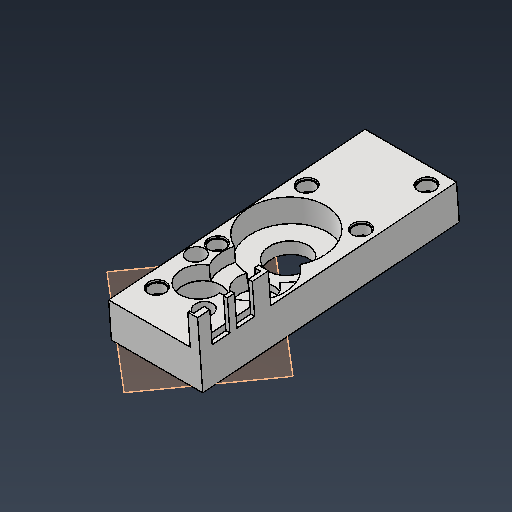
# Autodesk Inventor part: Right_gearbox
Saved by Autodesk Inventor 2026.2 (Build 302298010, 298A)
## iProperties
Created: 2026-04-04
Part Number: Right_gearbox
Material: Generic
Document SubType Name: Modeling
Designer: szymo
Density: 1 g/cm^3
Appearance: Default
Author: szymo
Autodesk Inventor part; units mm, degrees
(part 1 of 2)
ref_plane "YZ Plane" through (0, 0, 0) normal (1, 0, 0) x (0, 1, 0)
ref_plane "XZ Plane" through (0, 0, 0) normal (0, 1, 0) x (-1, 0, 0)
ref_plane "XY Plane" through (0, 0, 0) normal (0, 0, 1) x (1, 0, 0)
ref_plane "Work Plane1" through (-23.709139, -17.243721, 13.989977) normal (0, 0.9970894, 0.0762418) x (-1, 0, 0)
sketch "Sketch1" plane through (-23.709139, -17.243721, 13.989977) normal (0, 0.9970894, 0.0762418) x (-1, 0, 0)
  line L0 (0, -0.624975) -> (23.2, -0.624975)
  line L1 (23.2, -0.624975) -> (23.2, -65.920816)
  line L2 (23.2, -65.920816) -> (0, -65.920816)
  line L3 (0, -65.920816) -> (0, -0.624975)
  circle A0 centre (9.208398, -23.610194) radius 8 construction
  circle A1 centre (13, -35.626174) radius 9.6 construction
  circle A2 centre (9.208398, -23.610194) radius 8.4
  circle A3 centre (13, -35.626174) radius 10
  circle A4 centre (9.208398, -23.610194) radius 4.2 construction
  circle A5 centre (9.208398, -23.610194) radius 4.6
  circle A6 centre (14.459131, -15.124975) radius 1.15
  circle A7 centre (14.459131, -15.124975) radius 5
  circle A8 centre (14.5, -15.124975) radius 13.85 construction
  circle A9 centre (14.5, -55.920816) radius 14.5 construction
  circle A10 centre (14.5, -15.124975) radius 14.5 construction
  line L4 (19.165073, -50.048244) -> (22.270069, -47.442843)
  arc A11 (24.198432, -49.740976) -> (22.270069, -47.442843) centre (14.5, -55.920816) ccw
  line L5 (24.198432, -49.740976) -> (21.093435, -52.346377)
  arc A12 (21.093435, -52.346377) -> (19.165073, -50.048244) centre (14.5, -55.920816) ccw
  arc A13 (4.801568, -62.100655) -> (6.729931, -64.398789) centre (14.5, -55.920816) ccw
  line L6 (4.801568, -62.100655) -> (7.906565, -59.495254)
  arc A14 (7.906565, -59.495254) -> (9.834927, -61.793387) centre (14.5, -55.920816) ccw
  line L7 (9.834927, -61.793387) -> (6.729931, -64.398789)
  circle A15 centre (14.5, -55.920816) radius 5
  circle A16 centre (14.5, -55.920816) radius 13.85
  line L8 (20.703236, -53.979201) -> (25.489059, -49.963418)
  arc A17 (25.489059, -49.963418) -> (22.275121, -46.133196) centre (14.5, -55.920816) ccw
  line L9 (22.275121, -46.133196) -> (17.489298, -50.148979)
  arc A18 (20.703236, -53.979201) -> (17.489298, -50.148979) centre (14.5, -55.920816) ccw
  arc A19 (3.510941, -61.878213) -> (6.724879, -65.708435) centre (14.5, -55.920816) ccw
  line L10 (3.510941, -61.878213) -> (8.296764, -57.86243)
  arc A20 (8.296764, -57.86243) -> (11.510702, -61.692652) centre (14.5, -55.920816) ccw
  line L11 (11.510702, -61.692652) -> (6.724879, -65.708435)
  line L12 (6.724879, -65.708435) -> (6.724879, -65.920816)
  line L13 (11.510702, -61.692652) -> (23.2, -61.692652)
  arc A21 (20.63224, -38.75849) -> (22.059739, -38.801252) centre (21.52446, -32.822118) ccw
  arc A22 (22.059739, -38.801252) -> (22.213494, -38.322751) centre (13, -35.626174) ccw
  arc A23 (22.213494, -38.322751) -> (21.028277, -37.525981) centre (18.295517, -42.87094) ccw
  arc A24 (21.028277, -37.525981) -> (21.116703, -37.10321) centre (13, -35.626174) ccw
  arc A25 (21.116703, -37.10321) -> (22.521898, -36.848243) centre (20.755184, -31.111058) ccw
  arc A26 (22.521898, -36.848243) -> (22.572807, -36.348231) centre (13, -35.626174) ccw
  arc A27 (22.572807, -36.348231) -> (21.247832, -35.815293) centre (19.686069, -41.611625) ccw
  arc A28 (21.247832, -35.815293) -> (21.246426, -35.383375) centre (13, -35.626174) ccw
  arc A29 (21.246426, -35.383375) -> (22.567904, -34.841824) centre (19.64697, -29.597331) ccw
  arc A30 (22.567904, -34.841824) -> (22.513742, -34.342154) centre (13, -35.626174) ccw
  arc A31 (22.513742, -34.342154) -> (21.106917, -34.096339) centre (20.784408, -40.090717) ccw
  arc A32 (21.106917, -34.096339) -> (21.015742, -33.674153) centre (13, -35.626174) ccw
  arc A33 (21.015742, -33.674153) -> (22.195747, -32.869685) centre (18.248251, -28.347093) ccw
  arc A34 (22.195747, -32.869685) -> (22.038882, -32.392195) centre (13, -35.626174) ccw
  arc A35 (22.038882, -32.392195) -> (20.611691, -32.444247) centre (21.54253, -38.374686) ccw
  arc A36 (20.611691, -32.444247) -> (20.434731, -32.050243) centre (13, -35.626174) ccw
  arc A37 (20.434731, -32.050243) -> (21.421692, -31.018018) centre (16.620158, -27.414986) ccw
  arc A38 (21.421692, -31.018018) -> (21.168978, -30.583576) centre (13, -35.626174) ccw
  arc A39 (21.168978, -30.583576) -> (19.783798, -30.93122) centre (21.927304, -36.538533) ccw
  arc A40 (19.783798, -30.93122) -> (19.528786, -30.582618) centre (13, -35.626174) ccw
  arc A41 (19.528786, -30.582618) -> (20.279568, -29.367749) centre (14.833847, -26.841747) ccw
  arc A42 (20.279568, -29.367749) -> (19.942051, -28.995342) centre (13, -35.626174) ccw
  arc A43 (19.942051, -28.995342) -> (18.65942, -29.623385) centre (21.921911, -34.662505) ccw
  arc A44 (18.65942, -29.623385) -> (18.337502, -29.335421) centre (13, -35.626174) ccw
  arc A45 (18.337502, -29.335421) -> (18.819293, -27.991003) centre (12.967388, -26.652429) ccw
  arc A46 (18.819293, -27.991003) -> (18.411724, -27.696908) centre (13, -35.626174) ccw
  arc A47 (18.411724, -27.696908) -> (17.287698, -28.577901) centre (21.526587, -32.828594) ccw
  arc A48 (17.287698, -28.577901) -> (16.912944, -28.36316) centre (13, -35.626174) ccw
  arc A49 (16.912944, -28.36316) -> (17.104686, -26.947951) centre (11.102354, -26.855308) ccw
  arc A50 (17.104686, -26.947951) -> (16.644878, -26.745021) centre (13, -35.626174) ccw
  arc A51 (16.644878, -26.745021) -> (15.728583, -27.84046) centre (20.758611, -31.11695) ccw
  arc A52 (15.728583, -27.84046) -> (15.317371, -27.708327) centre (13, -35.626174) ccw
  arc A53 (15.317371, -27.708327) -> (15.210685, -26.284178) centre (9.320257, -27.441515) ccw
  arc A54 (15.210685, -26.284178) -> (14.718733, -26.181283) centre (13, -35.626174) ccw
  arc A55 (14.718733, -26.181283) -> (14.050216, -27.443292) centre (19.651547, -29.602382) ccw
  arc A56 (14.050216, -27.443292) -> (13.620518, -27.399543) centre (13, -35.626174) ccw
  arc A57 (13.620518, -27.399543) -> (13.220066, -26.028696) centre (7.698982, -28.385431) ccw
  arc A58 (13.220066, -26.028696) -> (12.717471, -26.030332) centre (13, -35.626174) ccw
  arc A59 (12.717471, -26.030332) -> (12.32595, -27.403756) centre (18.253778, -28.351081) ccw
  arc A60 (12.32595, -27.403756) -> (11.896546, -27.450301) centre (13, -35.626174) ccw
  arc A61 (11.896546, -27.450301) -> (11.219829, -26.19267) centre (6.309387, -29.645802) ccw
  arc A62 (11.219829, -26.19267) -> (10.728557, -26.298765) centre (13, -35.626174) ccw
  arc A63 (10.728557, -26.298765) -> (10.631143, -27.723578) centre (16.626394, -27.417738) ccw
  arc A64 (10.631143, -27.723578) -> (10.220799, -27.858385) centre (13, -35.626174) ccw
  arc A65 (10.220799, -27.858385) -> (9.297395, -26.768933) centre (5.212203, -31.167544) ccw
  arc A66 (9.297395, -26.768933) -> (8.838917, -26.974851) centre (13, -35.626174) ccw
  arc A67 (8.838917, -26.974851) -> (9.039866, -28.388782) centre (14.840518, -26.843142) ccw
  arc A68 (9.039866, -28.388782) -> (8.666517, -28.605958) centre (13, -35.626174) ccw
  arc A69 (8.666517, -28.605958) -> (7.536781, -27.7323) centre (4.455384, -32.88415) ccw
  arc A70 (7.536781, -27.7323) -> (7.131135, -28.029041) centre (13, -35.626174) ccw
  arc A71 (7.131135, -28.029041) -> (7.621666, -29.370294) centre (12.974204, -26.652407) ccw
  arc A72 (7.621666, -29.370294) -> (7.301629, -29.660348) centre (13, -35.626174) ccw
  arc A73 (7.301629, -29.660348) -> (6.014937, -29.040667) centre (4.072006, -34.720595) ccw
  arc A74 (6.014937, -29.040667) -> (5.679851, -29.415262) centre (13, -35.626174) ccw
  arc A75 (5.679851, -29.415262) -> (6.438525, -30.625219) centre (11.109017, -26.853869) ccw
  arc A76 (6.438525, -30.625219) -> (6.185788, -30.975474) centre (13, -35.626174) ccw
  arc A77 (6.185788, -30.975474) -> (4.798374, -30.636852) centre (4.078824, -36.596619) ccw
  arc A78 (4.798374, -30.636852) -> (4.548493, -31.07293) centre (13, -35.626174) ccw
  arc A79 (4.548493, -31.07293) -> (5.542152, -32.098709) centre (9.326474, -27.438722) ccw
  arc A80 (5.542152, -32.098709) -> (5.36776, -32.493857) centre (13, -35.626174) ccw
  arc A81 (5.36776, -32.493857) -> (3.940261, -32.451095) centre (4.47554, -38.430229) ccw
  arc A82 (3.940261, -32.451095) -> (3.786506, -32.929596) centre (13, -35.626174) ccw
  arc A83 (3.786506, -32.929596) -> (4.971723, -33.726366) centre (7.704483, -28.381407) ccw
  arc A84 (4.971723, -33.726366) -> (4.883297, -34.149138) centre (13, -35.626174) ccw
  arc A85 (4.883297, -34.149138) -> (3.478102, -34.404104) centre (5.244816, -40.141289) ccw
  arc A86 (3.478102, -34.404104) -> (3.427193, -34.904116) centre (13, -35.626174) ccw
  arc A87 (3.427193, -34.904116) -> (4.752168, -35.437054) centre (6.313931, -29.640722) ccw
  arc A88 (4.752168, -35.437054) -> (4.753574, -35.868972) centre (13, -35.626174) ccw
  arc A89 (4.753574, -35.868972) -> (3.432096, -36.410523) centre (6.35303, -41.655016) ccw
  arc A90 (3.432096, -36.410523) -> (3.486258, -36.910193) centre (13, -35.626174) ccw
  arc A91 (3.486258, -36.910193) -> (4.893083, -37.156008) centre (5.215592, -31.161631) ccw
  arc A92 (4.893083, -37.156008) -> (4.984258, -37.578194) centre (13, -35.626174) ccw
  arc A93 (4.984258, -37.578194) -> (3.804253, -38.382662) centre (7.751749, -42.905254) ccw
  arc A94 (3.804253, -38.382662) -> (3.961118, -38.860153) centre (13, -35.626174) ccw
  arc A95 (3.961118, -38.860153) -> (5.388309, -38.8081) centre (4.45747, -32.877661) ccw
  arc A96 (5.388309, -38.8081) -> (5.565269, -39.202104) centre (13, -35.626174) ccw
  arc A97 (5.565269, -39.202104) -> (4.578308, -40.234329) centre (9.379842, -43.837361) ccw
  arc A98 (4.578308, -40.234329) -> (4.831022, -40.668771) centre (13, -35.626174) ccw
  arc A99 (4.831022, -40.668771) -> (6.216202, -40.321127) centre (4.072696, -34.713814) ccw
  arc A100 (6.216202, -40.321127) -> (6.471214, -40.669729) centre (13, -35.626174) ccw
  arc A101 (6.471214, -40.669729) -> (5.720432, -41.884598) centre (11.166153, -44.4106) ccw
  arc A102 (5.720432, -41.884598) -> (6.057949, -42.257005) centre (13, -35.626174) ccw
  arc A103 (6.057949, -42.257005) -> (7.34058, -41.628962) centre (4.078089, -36.589842) ccw
  arc A104 (7.34058, -41.628962) -> (7.662498, -41.916926) centre (13, -35.626174) ccw
  arc A105 (7.662498, -41.916926) -> (7.180707, -43.261344) centre (13.032612, -44.599918) ccw
  arc A106 (7.180707, -43.261344) -> (7.588276, -43.555439) centre (13, -35.626174) ccw
  arc A107 (7.588276, -43.555439) -> (8.712302, -42.674446) centre (4.473413, -38.423753) ccw
  arc A108 (8.712302, -42.674446) -> (9.087056, -42.889187) centre (13, -35.626174) ccw
  arc A109 (9.087056, -42.889187) -> (8.895314, -44.304396) centre (14.897646, -44.397039) ccw
  arc A110 (8.895314, -44.304396) -> (9.355122, -44.507326) centre (13, -35.626174) ccw
  arc A111 (9.355122, -44.507326) -> (10.271417, -43.411887) centre (5.241389, -40.135397) ccw
  arc A112 (10.271417, -43.411887) -> (10.682629, -43.54402) centre (13, -35.626174) ccw
  arc A113 (10.682629, -43.54402) -> (10.789315, -44.968169) centre (16.679743, -43.810832) ccw
  arc A114 (10.789315, -44.968169) -> (11.281267, -45.071064) centre (13, -35.626174) ccw
  arc A115 (11.281267, -45.071064) -> (11.949784, -43.809055) centre (6.348453, -41.649966) ccw
  arc A116 (11.949784, -43.809055) -> (12.379482, -43.852804) centre (13, -35.626174) ccw
  arc A117 (12.379482, -43.852804) -> (12.779934, -45.223651) centre (18.301018, -42.866916) ccw
  arc A118 (12.779934, -45.223651) -> (13.282529, -45.222015) centre (13, -35.626174) ccw
  arc A119 (13.282529, -45.222015) -> (13.67405, -43.848591) centre (7.746222, -42.901266) ccw
  arc A120 (13.67405, -43.848591) -> (14.103454, -43.802046) centre (13, -35.626174) ccw
  arc A121 (14.103454, -43.802046) -> (14.780171, -45.059677) centre (19.690613, -41.606545) ccw
  arc A122 (14.780171, -45.059677) -> (15.271443, -44.953582) centre (13, -35.626174) ccw
  arc A123 (15.271443, -44.953582) -> (15.368857, -43.528769) centre (9.373606, -43.834609) ccw
  arc A124 (15.368857, -43.528769) -> (15.779201, -43.393962) centre (13, -35.626174) ccw
  arc A125 (15.779201, -43.393962) -> (16.702605, -44.483414) centre (20.787797, -40.084803) ccw
  arc A126 (16.702605, -44.483414) -> (17.161083, -44.277496) centre (13, -35.626174) ccw
  arc A127 (17.161083, -44.277496) -> (16.960134, -42.863565) centre (11.159482, -44.409205) ccw
  arc A128 (16.960134, -42.863565) -> (17.333483, -42.646389) centre (13, -35.626174) ccw
  arc A129 (17.333483, -42.646389) -> (18.463219, -43.520047) centre (21.544616, -38.368197) ccw
  arc A130 (18.463219, -43.520047) -> (18.868865, -43.223306) centre (13, -35.626174) ccw
  arc A131 (18.868865, -43.223306) -> (18.378334, -41.882053) centre (13.025796, -44.59994) ccw
  arc A132 (18.378334, -41.882053) -> (18.698371, -41.591999) centre (13, -35.626174) ccw
  arc A133 (18.698371, -41.591999) -> (19.985063, -42.21168) centre (21.927994, -36.531752) ccw
  arc A134 (19.985063, -42.21168) -> (20.320149, -41.837085) centre (13, -35.626174) ccw
  arc A135 (20.320149, -41.837085) -> (19.561475, -40.627128) centre (14.890983, -44.398478) ccw construction
  arc A136 (19.561475, -40.627128) -> (19.814212, -40.276874) centre (13, -35.626174) ccw
  arc A137 (19.814212, -40.276874) -> (21.201626, -40.615495) centre (21.921176, -34.655728) ccw
  arc A138 (21.201626, -40.615495) -> (21.451507, -40.179417) centre (13, -35.626174) ccw
  arc A139 (21.451507, -40.179417) -> (20.457848, -39.153638) centre (16.673526, -43.813625) ccw
  arc A140 (20.457848, -39.153638) -> (20.63224, -38.75849) centre (13, -35.626174) ccw
  circle A141 centre (13, -35.626174) radius 5
  circle A142 centre (9.208398, -23.610194) radius 1.25
  arc A143 (5.40627, -25.394522) -> (6.808495, -25.147389) centre (5.476375, -21.690633) ccw
  arc A144 (6.808495, -25.147389) -> (7.029671, -25.447488) centre (9.208398, -23.610194) ccw
  arc A145 (7.029671, -25.447488) -> (6.378522, -26.713709) centre (9.937158, -27.743186) ccw
  arc A146 (6.378522, -26.713709) -> (6.807822, -27.056531) centre (9.208398, -23.610194) ccw
  arc A147 (6.807822, -27.056531) -> (7.898619, -26.141395) centre (5.01659, -23.813817) ccw
  arc A148 (7.898619, -26.141395) -> (8.240212, -26.290701) centre (9.208398, -23.610194) ccw
  arc A149 (8.240212, -26.290701) -> (8.309411, -27.712855) centre (11.906019, -26.82509) ccw
  arc A150 (8.309411, -27.712855) -> (8.852607, -27.795097) centre (9.208398, -23.610194) ccw
  arc A151 (8.852607, -27.795097) -> (9.339696, -26.457168) centre (5.679997, -25.88244) ccw
  arc A152 (9.339696, -26.457168) -> (9.710178, -26.415674) centre (9.208398, -23.610194) ccw
  arc A153 (9.710178, -26.415674) -> (10.481183, -27.612696) centre (13.152054, -25.045566) ccw
  arc A154 (10.481183, -27.612696) -> (10.992725, -27.412322) centre (9.208398, -23.610194) ccw
  arc A155 (10.992725, -27.412322) -> (10.745593, -26.010097) centre (7.288836, -27.342217) ccw
  arc A156 (10.745593, -26.010097) -> (11.045692, -25.788921) centre (9.208398, -23.610194) ccw
  arc A157 (11.045692, -25.788921) -> (12.311913, -26.44007) centre (13.34139, -22.881434) ccw
  arc A158 (12.311913, -26.44007) -> (12.654735, -26.01077) centre (9.208398, -23.610194) ccw
  arc A159 (12.654735, -26.01077) -> (11.739599, -24.919974) centre (9.41202, -27.802002) ccw
  arc A160 (11.739599, -24.919974) -> (11.888905, -24.57838) centre (9.208398, -23.610194) ccw
  arc A161 (11.888905, -24.57838) -> (13.311058, -24.509181) centre (12.423294, -20.912574) ccw
  arc A162 (13.311058, -24.509181) -> (13.393301, -23.965986) centre (9.208398, -23.610194) ccw
  arc A163 (13.393301, -23.965986) -> (12.055372, -23.478896) centre (11.480644, -27.138595) ccw
  arc A164 (12.055372, -23.478896) -> (12.013878, -23.108415) centre (9.208398, -23.610194) ccw
  arc A165 (12.013878, -23.108415) -> (13.210899, -22.337409) centre (10.643769, -19.666538) ccw
  arc A166 (13.210899, -22.337409) -> (13.010526, -21.825867) centre (9.208398, -23.610194) ccw
  arc A167 (13.010526, -21.825867) -> (11.608301, -22.073) centre (12.940421, -25.529756) ccw
  arc A168 (11.608301, -22.073) -> (11.387125, -21.772901) centre (9.208398, -23.610194) ccw
  arc A169 (11.387125, -21.772901) -> (12.038273, -20.50668) centre (8.479638, -19.477202) ccw
  arc A170 (12.038273, -20.50668) -> (11.608973, -20.163858) centre (9.208398, -23.610194) ccw
  arc A171 (11.608973, -20.163858) -> (10.518177, -21.078994) centre (13.400206, -23.406572) ccw
  arc A172 (10.518177, -21.078994) -> (10.176584, -20.929688) centre (9.208398, -23.610194) ccw
  arc A173 (10.176584, -20.929688) -> (10.107385, -19.507534) centre (6.510777, -20.395298) ccw
  arc A174 (10.107385, -19.507534) -> (9.564189, -19.425291) centre (9.208398, -23.610194) ccw
  arc A175 (9.564189, -19.425291) -> (9.0771, -20.76322) centre (12.736799, -21.337949) ccw
  arc A176 (9.0771, -20.76322) -> (8.706618, -20.804715) centre (9.208398, -23.610194) ccw
  arc A177 (8.706618, -20.804715) -> (7.935613, -19.607693) centre (5.264742, -22.174823) ccw
  arc A178 (7.935613, -19.607693) -> (7.42407, -19.808067) centre (9.208398, -23.610194) ccw
  arc A179 (7.42407, -19.808067) -> (7.671203, -21.210292) centre (11.12796, -19.878171) ccw
  arc A180 (7.671203, -21.210292) -> (7.371104, -21.431467) centre (9.208398, -23.610194) ccw
  arc A181 (7.371104, -21.431467) -> (6.104883, -20.780319) centre (5.075406, -24.338955) ccw
  arc A182 (6.104883, -20.780319) -> (5.762061, -21.209619) centre (9.208398, -23.610194) ccw
  arc A183 (5.762061, -21.209619) -> (6.677197, -22.300415) centre (9.004776, -19.418387) ccw
  arc A184 (6.677197, -22.300415) -> (6.527891, -22.642008) centre (9.208398, -23.610194) ccw
  arc A185 (6.527891, -22.642008) -> (5.105737, -22.711208) centre (5.993502, -26.307815) ccw
  arc A186 (5.105737, -22.711208) -> (5.023495, -23.254403) centre (9.208398, -23.610194) ccw
  arc A187 (5.023495, -23.254403) -> (6.361424, -23.741493) centre (6.936152, -20.081794) ccw
  arc A188 (6.361424, -23.741493) -> (6.402918, -24.111974) centre (9.208398, -23.610194) ccw
  arc A189 (6.402918, -24.111974) -> (5.205896, -24.882979) centre (7.773027, -27.553851) ccw
  arc A190 (5.205896, -24.882979) -> (5.40627, -25.394522) centre (9.208398, -23.610194) ccw
  circle A191 centre (9.208398, -23.610194) radius 1.25
  arc A192 (17.179273, -22.928177) -> (16.018307, -22.666389) centre (15.506202, -27.642647) ccw
  arc A193 (16.018307, -22.666389) -> (15.959579, -22.311279) centre (9.208398, -23.610194) ccw
  arc A194 (15.959579, -22.311279) -> (16.974447, -21.689654) centre (13.872622, -17.764852) ccw
  arc A195 (16.974447, -21.689654) -> (16.863291, -21.285842) centre (9.208398, -23.610194) ccw
  arc A196 (16.863291, -21.285842) -> (15.673266, -21.271154) centre (16.206974, -26.245141) ccw
  arc A197 (15.673266, -21.271154) -> (15.54199, -20.936014) centre (9.208398, -23.610194) ccw
  arc A198 (15.54199, -20.936014) -> (16.405438, -20.11697) centre (12.555382, -16.92284) ccw
  arc A199 (16.405438, -20.11697) -> (16.212753, -19.745093) centre (9.208398, -23.610194) ccw
  arc A200 (16.212753, -19.745093) -> (15.045679, -19.978146) centre (16.601875, -24.732476) ccw
  arc A201 (15.045679, -19.978146) -> (14.847592, -19.677624) centre (9.208398, -23.610194) ccw
  arc A202 (14.847592, -19.677624) -> (15.521883, -18.696957) centre (11.091863, -16.373097) ccw
  arc A203 (15.521883, -18.696957) -> (15.256092, -18.373268) centre (9.208398, -23.610194) ccw
  arc A204 (15.256092, -18.373268) -> (14.162975, -18.843876) centre (16.673645, -23.170761) ccw
  arc A205 (14.162975, -18.843876) -> (13.906735, -18.591106) centre (9.208398, -23.610194) ccw
  arc A206 (13.906735, -18.591106) -> (14.362399, -17.491675) centre (9.546028, -16.139651) ccw
  arc A207 (14.362399, -17.491675) -> (14.035117, -17.230321) centre (9.208398, -23.610194) ccw
  arc A208 (14.035117, -17.230321) -> (13.063732, -17.917917) centre (16.419148, -21.628251) ccw
  arc A209 (13.063732, -17.917917) -> (12.760538, -17.723945) centre (9.208398, -23.610194) ccw
  arc A210 (12.760538, -17.723945) -> (12.97766, -16.553803) centre (7.985437, -16.232703) ccw
  arc A211 (12.97766, -16.553803) -> (12.603191, -16.366205) centre (9.208398, -23.610194) ccw
  arc A212 (12.603191, -16.366205) -> (11.795993, -17.240738) centre (15.849507, -20.172362) ccw
  arc A213 (11.795993, -17.240738) -> (11.459095, -17.114043) centre (9.208398, -23.610194) ccw
  arc A214 (11.459095, -17.114043) -> (11.428186, -15.924328) centre (6.478294, -16.648187) ccw
  arc A215 (11.428186, -15.924328) -> (11.022897, -15.818687) centre (9.208398, -23.610194) ccw
  arc A216 (11.022897, -15.818687) -> (10.415163, -16.841935) centre (14.989617, -18.866723) ccw
  arc A217 (10.415163, -16.841935) -> (10.059286, -16.788053) centre (9.208398, -23.610194) ccw
  arc A218 (10.059286, -16.788053) -> (9.781697, -15.630763) centre (5.090471, -17.367944) ccw
  arc A219 (9.781697, -15.630763) -> (9.3633, -15.611694) centre (9.208398, -23.610194) ccw
  arc A220 (9.3633, -15.611694) -> (8.981592, -16.738937) centre (13.87706, -17.768396) ccw
  arc A221 (8.981592, -16.738937) -> (8.622289, -16.760224) centre (9.208398, -23.610194) ccw
  arc A222 (8.622289, -16.760224) -> (8.110152, -15.685937) centre (3.882621, -18.360517) ccw
  arc A223 (8.110152, -15.685937) -> (7.696933, -15.754275) centre (9.208398, -23.610194) ccw
  arc A224 (7.696933, -15.754275) -> (7.557934, -16.936246) centre (12.560461, -16.925384) ccw
  arc A225 (7.557934, -16.936246) -> (7.210908, -17.031771) centre (9.208398, -23.610194) ccw
  arc A226 (7.210908, -17.031771) -> (6.486605, -16.087439) centre (2.907532, -19.582526) ccw
  arc A227 (6.486605, -16.087439) -> (6.096625, -16.240197) centre (9.208398, -23.610194) ccw
  arc A228 (6.096625, -16.240197) -> (6.206408, -17.425238) centre (11.09736, -16.37453) ccw
  arc A229 (6.206408, -17.425238) -> (5.886827, -17.590827) centre (9.208398, -23.610194) ccw
  arc A230 (5.886827, -17.590827) -> (4.982014, -16.817722) centre (2.207822, -20.980564) ccw
  arc A231 (4.982014, -16.817722) -> (4.632316, -17.048223) centre (9.208398, -23.610194) ccw
  arc A232 (4.632316, -17.048223) -> (4.986084, -18.184543) centre (9.551702, -16.139909) ccw
  arc A233 (4.986084, -18.184543) -> (4.707914, -18.412958) centre (9.208398, -23.610194) ccw
  arc A234 (4.707914, -18.412958) -> (3.662136, -17.844868) centre (1.81407, -22.493529) ccw
  arc A235 (3.662136, -17.844868) -> (3.368003, -18.143039) centre (9.208398, -23.610194) ccw
  arc A236 (3.368003, -18.143039) -> (3.950295, -19.180975) centre (7.991041, -16.231776) ccw
  arc A237 (3.950295, -19.180975) -> (3.725694, -19.462233) centre (9.208398, -23.610194) ccw
  arc A238 (3.725694, -19.462233) -> (2.584657, -19.123987) centre (1.743487, -24.055298) ccw
  arc A239 (2.584657, -19.123987) -> (2.358945, -19.476795) centre (9.208398, -23.610194) ccw
  arc A240 (2.358945, -19.476795) -> (3.144311, -20.370985) centre (6.483583, -16.646115) ccw
  arc A241 (3.144311, -20.370985) -> (2.983095, -20.692794) centre (9.208398, -23.610194) ccw
  arc A242 (2.983095, -20.692794) -> (1.796667, -20.599175) centre (1.999155, -25.597614) ccw
  arc A243 (1.796667, -20.599175) -> (1.649239, -20.991201) centre (9.208398, -23.610194) ccw
  arc A244 (1.649239, -20.991201) -> (2.603356, -21.702564) centre (5.095213, -17.364818) ccw
  arc A245 (2.603356, -21.702564) -> (2.512571, -22.05086) centre (9.208398, -23.610194) ccw
  arc A246 (2.512571, -22.05086) -> (1.332604, -22.205958) centre (2.569902, -27.05307) ccw
  arc A247 (1.332604, -22.205958) -> (1.269906, -22.62007) centre (9.208398, -23.610194) ccw
  arc A248 (1.269906, -22.62007) -> (2.351074, -23.117516) centre (3.886609, -18.356473) ccw
  arc A249 (2.351074, -23.117516) -> (2.334687, -23.477076) centre (9.208398, -23.610194) ccw
  arc A250 (2.334687, -23.477076) -> (1.212752, -23.874114) centre (3.430783, -28.358056) ccw
  arc A251 (1.212752, -23.874114) -> (1.237523, -24.292212) centre (9.208398, -23.610194) ccw
  arc A252 (1.237523, -24.292212) -> (2.398489, -24.554) centre (2.910593, -19.577742) ccw
  arc A253 (2.398489, -24.554) -> (2.457217, -24.909109) centre (9.208398, -23.610194) ccw
  arc A254 (2.457217, -24.909109) -> (1.442348, -25.530735) centre (4.544174, -29.455537) ccw
  arc A255 (1.442348, -25.530735) -> (1.553505, -25.934546) centre (9.208398, -23.610194) ccw
  arc A256 (1.553505, -25.934546) -> (2.74353, -25.949235) centre (2.209821, -20.975248) ccw
  arc A257 (2.74353, -25.949235) -> (2.874806, -26.284374) centre (9.208398, -23.610194) ccw
  arc A258 (2.874806, -26.284374) -> (2.011358, -27.103419) centre (5.861413, -30.297549) ccw
  arc A259 (2.011358, -27.103419) -> (2.204043, -27.475295) centre (9.208398, -23.610194) ccw
  arc A260 (2.204043, -27.475295) -> (3.371117, -27.242243) centre (1.814921, -22.487913) ccw
  arc A261 (3.371117, -27.242243) -> (3.569203, -27.542765) centre (9.208398, -23.610194) ccw
  arc A262 (3.569203, -27.542765) -> (2.894913, -28.523432) centre (7.324932, -30.847292) ccw
  arc A263 (2.894913, -28.523432) -> (3.160704, -28.847121) centre (9.208398, -23.610194) ccw
  arc A264 (3.160704, -28.847121) -> (4.253821, -28.376513) centre (1.743151, -24.049628) ccw
  arc A265 (4.253821, -28.376513) -> (4.510061, -28.629283) centre (9.208398, -23.610194) ccw
  arc A266 (4.510061, -28.629283) -> (4.054397, -29.728714) centre (8.870768, -31.080738) ccw
  arc A267 (4.054397, -29.728714) -> (4.381679, -29.990068) centre (9.208398, -23.610194) ccw
  arc A268 (4.381679, -29.990068) -> (5.353064, -29.302472) centre (1.997648, -25.592138) ccw
  arc A269 (5.353064, -29.302472) -> (5.656258, -29.496443) centre (9.208398, -23.610194) ccw
  arc A270 (5.656258, -29.496443) -> (5.439136, -30.666586) centre (10.431359, -30.987686) ccw
  arc A271 (5.439136, -30.666586) -> (5.813605, -30.854184) centre (9.208398, -23.610194) ccw
  arc A272 (5.813605, -30.854184) -> (6.620803, -29.979651) centre (2.567289, -27.048027) ccw
  arc A273 (6.620803, -29.979651) -> (6.957701, -30.106346) centre (9.208398, -23.610194) ccw
  arc A274 (6.957701, -30.106346) -> (6.98861, -31.296061) centre (11.938501, -30.572202) ccw
  arc A275 (6.98861, -31.296061) -> (7.393899, -31.401702) centre (9.208398, -23.610194) ccw
  arc A276 (7.393899, -31.401702) -> (8.001633, -30.378454) centre (3.427179, -28.353666) ccw
  arc A277 (8.001633, -30.378454) -> (8.35751, -30.432336) centre (9.208398, -23.610194) ccw
  arc A278 (8.35751, -30.432336) -> (8.635099, -31.589626) centre (13.326325, -29.852445) ccw
  arc A279 (8.635099, -31.589626) -> (9.053496, -31.608695) centre (9.208398, -23.610194) ccw
  arc A280 (9.053496, -31.608695) -> (9.435204, -30.481452) centre (4.539735, -29.451993) ccw
  arc A281 (9.435204, -30.481452) -> (9.794507, -30.460165) centre (9.208398, -23.610194) ccw
  arc A282 (9.794507, -30.460165) -> (10.306644, -31.534452) centre (14.534175, -28.859872) ccw
  arc A283 (10.306644, -31.534452) -> (10.719863, -31.466114) centre (9.208398, -23.610194) ccw
  arc A284 (10.719863, -31.466114) -> (10.858862, -30.284143) centre (5.856335, -30.295005) ccw
  arc A285 (10.858862, -30.284143) -> (11.205888, -30.188618) centre (9.208398, -23.610194) ccw
  arc A286 (11.205888, -30.188618) -> (11.930191, -31.13295) centre (15.509264, -27.637863) ccw
  arc A287 (11.930191, -31.13295) -> (12.320171, -30.980192) centre (9.208398, -23.610194) ccw
  arc A288 (12.320171, -30.980192) -> (12.210388, -29.795151) centre (7.319436, -30.845859) ccw
  arc A289 (12.210388, -29.795151) -> (12.529969, -29.629562) centre (9.208398, -23.610194) ccw
  arc A290 (12.529969, -29.629562) -> (13.434782, -30.402667) centre (16.208974, -26.239825) ccw
  arc A291 (13.434782, -30.402667) -> (13.78448, -30.172166) centre (9.208398, -23.610194) ccw
  arc A292 (13.78448, -30.172166) -> (13.430712, -29.035846) centre (8.865094, -31.08048) ccw
  arc A293 (13.430712, -29.035846) -> (13.708882, -28.807431) centre (9.208398, -23.610194) ccw
  arc A294 (13.708882, -28.807431) -> (14.754659, -29.37552) centre (16.602725, -24.726859) ccw
  arc A295 (14.754659, -29.37552) -> (15.048792, -29.07735) centre (9.208398, -23.610194) ccw
  arc A296 (15.048792, -29.07735) -> (14.4665, -28.039414) centre (10.425755, -30.988613) ccw
  arc A297 (14.4665, -28.039414) -> (14.691102, -27.758156) centre (9.208398, -23.610194) ccw
  arc A298 (14.691102, -27.758156) -> (15.832139, -28.096402) centre (16.673309, -23.165091) ccw
  arc A299 (15.832139, -28.096402) -> (16.057851, -27.743594) centre (9.208398, -23.610194) ccw
  arc A300 (16.057851, -27.743594) -> (15.272485, -26.849404) centre (11.933213, -30.574274) ccw
  arc A301 (15.272485, -26.849404) -> (15.433701, -26.527595) centre (9.208398, -23.610194) ccw
  arc A302 (15.433701, -26.527595) -> (16.620129, -26.621214) centre (16.417641, -21.622775) ccw
  arc A303 (16.620129, -26.621214) -> (16.767556, -26.229187) centre (9.208398, -23.610194) ccw
  arc A304 (16.767556, -26.229187) -> (15.813439, -25.517825) centre (13.321582, -29.855571) ccw
  arc A305 (15.813439, -25.517825) -> (15.904225, -25.169529) centre (9.208398, -23.610194) ccw
  arc A306 (15.904225, -25.169529) -> (17.084191, -25.01443) centre (15.846894, -20.167319) ccw
  arc A307 (17.084191, -25.01443) -> (17.14689, -24.600319) centre (9.208398, -23.610194) ccw
  arc A308 (17.14689, -24.600319) -> (16.065722, -24.102873) centre (14.530186, -28.863916) ccw
  arc A309 (16.065722, -24.102873) -> (16.082109, -23.743313) centre (9.208398, -23.610194) ccw
  arc A310 (16.082109, -23.743313) -> (17.204043, -23.346275) centre (14.986013, -18.862333) ccw
  arc A311 (17.204043, -23.346275) -> (17.179273, -22.928177) centre (9.208398, -23.610194) ccw
  point P0 (23.2, -65.461045)
  point P1 (4.410688, -30.505264)
  point P2 (17.094606, -26.502896)
  point P3 (13.340279, -25.631965)
  point P4 (6.985214, -27.637284)
  point P5 (11.102341, -18.793206)
  point P6 (12.37974, -19.653164)
  point P7 (23.2, -45.144337)
  point P8 (4.917594, -65.920816)
  point P9 (23.2, -51.884167)
  point P10 (23.2, -46.945293)
  point P11 (11.076423, -25.812925)
  point P12 (10.997401, -25.828745)
  dimension "d0" = 0.4
  dimension "d1" = 0.4
  dimension "d3" = 0.2
  dimension "d108" = 0.4
  dimension "d125" = 4.5
  dimension "d126" = 1
  dimension "d127" = 1
  constraints: 20 end point, 8 point on circle, 7 centre point, 3 coincident, 3 perpendicular, 3 point on line, 2 parallel, 2 tangent, 1 horizontal, 15 other
  measures "d3" distance edge to line of A3 L1
  measures "d125" distance edge to line of A9 L2
  measures "d126" distance between parallel lines of L5 L8
  measures "d127" distance between parallel lines of L7 L11
ref_plane "Work Plane6" through (-57.598855, -15.421375, -20.139684) normal (0, 1, 0) x (-0.6427876, 0, 0.7660444)
ref_plane "Work Plane8" through (-57.598855, -16.714092, -20.48043) normal (0, 0.9970894, 0.0762418) x (-0.6427876, -0.0584046, 0.7638148)
extrude "Extrusion2" add sketch "Sketch1" against normal up to surface (2.1 mm away) contours L0 L1 A16 A3 A2 A7 L2 L3 | A16 A109 A108 A107 A106 A105 A104 A103 A102 A101 A100 A99 A98 A97 A96 A95 A94 A93 A92 A91 A90 A89 A88 A87 A86 A85 A84 A83 A82 A81 A80 A79 A78 A2 A141 A3 | A3 A2 A78 A79 A80 A81 A82 A83 A84 A85 A86 A87 A88 A89 A90 A91 A92 A93 A94 A95 A96 A97 A98 A99 A100 A101 A102 A103 A104 A105 A106 A107 A108 A109 A16 | A3 A268 A269 A270 A271 A77 A78 A2 | A2 A7 A219 A220 A221 A222 A223 A224 A225 A226 A227 A228 A229 A230 A231 A232 A233 A234 A235 A236 A237 A238 A239 A240 A241 A242 A243 A244 A245 A246 A247 A248 A249 A250 A251 A252 A253 A254 A255 A256 A257 A258 A259 A260 A261 A262 A263 A264 A265 A266 A267 A268 A3 | A3 A303 A304 A305 A306 A307 A308 A309 A310 A311 A192 A193 A194 A195 A196 A197 A198 A199 A7 A2 | A2 A50 A51 A300 A53 A301 A302 A303 A3 | A78 A77 A271 A272 A76 A75 A273 A274 A275 A276 A277 A278 A279 A280 A281 A282 A141 A2 | A268 A267 A266 A265 A264 A263 A262 A261 A260 A259 A258 A257 A256 A255 A254 A253 A252 A251 A250 A249 A248 A247 A246 A245 A244 A243 A242 A241 A240 A239 A238 A237 A236 A235 A234 A233 A232 A231 A230 A229 A228 A227 A226 A225 A224 A223 A222 A221 A220 A219 A7 A199 A198 A197 A196 A195 A194 A193 A192 A311 A310 A309 A308 A307 A306 A305 A304 A303 A3 A5 | A3 A5 A70 A71 A72 A73 A74 A75 A272 A77 A271 A270 A269 A268 | A2 A141 A288 A289 A290 A291 A292 A293 A294 A295 A296 A297 A298 A299 A300 A51 A50 | A303 A302 A301 A53 A54 A55 A56 A57 A58 A5 A3 | A282 A281 A280 A279 A278 A277 A276 A275 A274 A273 A272 A75 A74 A73 A72 A71 A70 A5 A69 A68 A67 A61 A60 A59 A58 A57 A56 A55 A54 A53 A301 A300 A52 A51 A299 A298 A297 A296 A295 A294 A293 A292 A291 A290 A289 A288 A141 A286 A285 A284 | A77 A272 A271 | A51 A52 A53 A300 | A284 A285 A286 A141 | A272 A75 A76 A77 | A5 A67 A68 A69 | A300 A301 A53 | A59 A60 A61 A5
extrude "Extrusion3" add sketch "Sketch1" along normal blind 1 contours L0 L1 A16 A3 A2 A7 L2 L3 | L1 A17 L9 A18 L8 L13 A20 L10 A19 L12 L2 A16 A3 | A16 A109 A108 A107 A106 A105 A104 A103 A102 A101 A100 A99 A98 A97 A96 A95 A94 A93 A92 A91 A90 A89 A88 A87 A86 A85 A84 A83 A82 A81 A80 A79 A78 A2 A141 A3 | A3 A16 A109 A110 A111 A112 A113 A114 A115 A116 A117 A118 A119 A120 A121 A122 A123 A124 A125 A126 A127 A128 A129 A130 A131 | A3 A2 A78 A79 A80 A81 A82 A83 A84 A85 A86 A87 A88 A89 A90 A91 A92 A93 A94 A95 A96 A97 A98 A99 A100 A101 A102 A103 A104 A105 A106 A107 A108 A109 A16 | A131 A130 A129 A128 A127 A126 A125 A124 A123 A122 A121 A120 A119 A118 A117 A116 A115 A114 A113 A112 A111 A110 A109 A16 | A3 A268 A269 A270 A271 A77 A78 A2 | A2 A7 A219 A220 A221 A222 A223 A224 A225 A226 A227 A228 A229 A230 A231 A232 A233 A234 A235 A236 A237 A238 A239 A240 A241 A242 A243 A244 A245 A246 A247 A248 A249 A250 A251 A252 A253 A254 A255 A256 A257 A258 A259 A260 A261 A262 A263 A264 A265 A266 A267 A268 A3 | A3 A303 A304 A305 A306 A307 A308 A309 A310 A311 A192 A193 A194 A195 A196 A197 A198 A199 A7 A2 | A2 A50 A51 A300 A53 A301 A302 A303 A3 | A78 A77 A271 A272 A76 A75 A273 A274 A275 A276 A277 A278 A279 A280 A281 A282 A141 A2 | A268 A267 A266 A265 A264 A263 A262 A261 A260 A259 A258 A257 A256 A255 A254 A253 A252 A251 A250 A249 A248 A247 A246 A245 A244 A243 A242 A241 A240 A239 A238 A237 A236 A235 A234 A233 A232 A231 A230 A229 A228 A227 A226 A225 A224 A223 A222 A221 A220 A219 A7 A199 A198 A197 A196 A195 A194 A193 A192 A311 A310 A309 A308 A307 A306 A305 A304 A303 A3 A5 | A3 A5 A70 A71 A72 A73 A74 A75 A272 A77 A271 A270 A269 A268 | A2 A141 A288 A289 A290 A291 A292 A293 A294 A295 A296 A297 A298 A299 A300 A51 A50 | A303 A302 A301 A53 A54 A55 A56 A57 A58 A5 A3 | A282 A281 A280 A279 A278 A277 A276 A275 A274 A273 A272 A75 A74 A73 A72 A71 A70 A5 A69 A68 A67 A61 A60 A59 A58 A57 A56 A55 A54 A53 A301 A300 A52 A51 A299 A298 A297 A296 A295 A294 A293 A292 A291 A290 A289 A288 A141 A286 A285 A284 | A77 A272 A271 | A51 A52 A53 A300 | A284 A285 A286 A141 | A272 A75 A76 A77 | A5 A67 A68 A69 | A300 A301 A53 | A59 A60 A61 A5
extrude "Extrusion4" add sketch "Sketch1" along normal blind 3.4 contours L0 L1 A16 A3 A2 A7 L2 L3 | L1 A17 L9 A18 L8 L13 A20 L10 A19 L12 L2 A16 A3 | A2 A7 A219 A220 A221 A222 A223 A224 A225 A226 A227 A228 A229 A230 A231 A232 A233 A234 A235 A236 A237 A238 A239 A240 A241 A242 A243 A244 A245 A246 A247 A248 A249 A250 A251 A252 A253 A254 A255 A256 A257 A258 A259 A260 A261 A262 A263 A264 A265 A266 A267 A268 A3 | A3 A303 A304 A305 A306 A307 A308 A309 A310 A311 A192 A193 A194 A195 A196 A197 A198 A199 A7 A2 | A268 A267 A266 A265 A264 A263 A262 A261 A260 A259 A258 A257 A256 A255 A254 A253 A252 A251 A250 A249 A248 A247 A246 A245 A244 A243 A242 A241 A240 A239 A238 A237 A236 A235 A234 A233 A232 A231 A230 A229 A228 A227 A226 A225 A224 A223 A222 A221 A220 A219 A7 A199 A198 A197 A196 A195 A194 A193 A192 A311 A310 A309 A308 A307 A306 A305 A304 A303 A3 A5